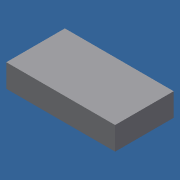
# Autodesk Inventor part: Part16
Saved by Autodesk Inventor 2014 (Build 180170000, 170)
## iProperties
Created: 2014-04-18
Part Number: Part16
Material: Generic
Document SubType Name: Modeling
Designer: Lefo
Density: 1 g/cm^3
Appearance: Default
Author: Lefo
Autodesk Inventor part; units mm, degrees
ref_plane "YZ Plane" through (0, 0, 0) normal (1, 0, 0) x (0, 1, 0)
ref_plane "XZ Plane" through (0, 0, 0) normal (0, 1, 0) x (-1, 0, 0)
ref_plane "XY Plane" through (0, 0, 0) normal (0, 0, 1) x (1, 0, 0)
sketch "Sketch1" plane through (0, 0, 0) normal (0, 1, 0) x (-1, 0, 0)
  line L0 (26, -14) -> (-26, -14)
  line L1 (-26, -14) -> (-26, 14)
  line L2 (-26, 14) -> (26, 14)
  line L3 (26, 14) -> (26, -14)
  line L4 (26, -14) -> (-26, 14) construction
  line L5 (-26, -14) -> (26, 14) construction
  point P0 (0, 0)
  dimension "d0" = 52
  dimension "d1" = 28
  constraints: 12 end point, 2 midpoint, 2 parallel, 1 horizontal, 1 perpendicular
  measures "d0" distance of L1.end L2.end
  measures "d1" distance of L0.end L1.end
extrude "Extrusion1" add sketch "Sketch1" along normal blind 11
body "Solid1"
